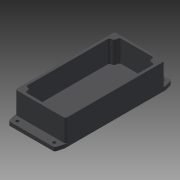
# Autodesk Inventor part: NEAMBoxLarge
Saved by Autodesk Inventor 2014 (Build 180170000, 170)
## iProperties
Created: 2015-04-18
Part Number: NEAMBoxLarge
Material: Generic
Document SubType Name: Modeling
Designer: Owner
Density: 1 g/cm^3
Appearance: Gray
Author: Owner
Autodesk Inventor part; units mm, degrees
ref_plane "YZ Plane" through (0, 0, 0) normal (1, 0, 0) x (0, 1, 0)
ref_plane "XZ Plane" through (0, 0, 0) normal (0, 1, 0) x (-1, 0, 0)
ref_plane "XY Plane" through (0, 0, 0) normal (0, 0, 1) x (1, 0, 0)
sketch "Sketch1" plane through (0, 0, 0) normal (0, 1, 0) x (-1, 0, 0)
  line L0 (-41.2899, 41.3823) -> (28.4387, 41.3823)
  line L1 (34.2779, 28.6823) -> (34.2779, -135.3255)
  line L2 (28.4387, -148.0255) -> (-41.2899, -148.0255)
  line L3 (-47.1291, -135.3255) -> (-47.1291, 28.6823)
  line L4 (-47.1291, 28.6823) -> (34.2779, 28.6823)
  line L5 (-47.1291, -135.3255) -> (34.2779, -135.3255)
  line L6 (34.2779, -135.3255) -> (31.5055, -145.6722)
  line L7 (-47.1291, -135.3255) -> (-44.3567, -145.6722)
  line L8 (-47.1291, 28.6823) -> (-44.3567, 39.0291)
  line L9 (34.2779, 28.6823) -> (31.5055, 39.0291)
  arc A0 (-44.3567, -145.6722) -> (-41.2899, -148.0255) centre (-41.2899, -144.8505) ccw
  arc A1 (28.4387, -148.0255) -> (31.5055, -145.6722) centre (28.4387, -144.8505) ccw
  arc A2 (31.5055, 39.0291) -> (28.4387, 41.3823) centre (28.4387, 38.2073) ccw
  arc A3 (-41.2899, 41.3823) -> (-44.3567, 39.0291) centre (-41.2899, 38.2073) ccw
  circle A4 centre (-36.423, -141.0151) radius 2.5019
  circle A5 centre (23.5718, -141.0151) radius 2.5019
  circle A6 centre (-36.423, 34.3719) radius 2.5019
  circle A7 centre (23.5718, 34.3719) radius 2.5019
  line L10 (-6.4256, 41.3823) -> (-6.4256, -148.0255) construction
  point P0 (0, 0)
  dimension "d2" = 12.7
  dimension "d3" = 12.7
  dimension "d4" = 15
  dimension "d5" = 15
  dimension "d6" = 15
  dimension "d7" = 81.407
  dimension "d8" = 189.4078
  dimension "d9" = 3.175
  dimension "d10" = 7.0104
  dimension "d11" = 7.0104
  dimension "d12" = 7.0104
  dimension "d13" = 7.0104
  dimension "d14" = 59.9948
  dimension "d15" = 59.9948
  dimension "d16" = 5.0038
  dimension "d17" = 5.0038
  dimension "d18" = 5.0038
  dimension "d19" = 5.0038
  dimension "d20" = 29.9974
  dimension "d21" = 29.9974
  constraints: 22 end point, 8 centre point, 8 point on circle, 8 tangent, 3 equal radius, 3 parallel, 3 perpendicular, 2 midpoint, 1 horizontal
  measures "d2" distance between parallel lines of L0 L4
  measures "d3" distance between parallel lines of L2 L5
  measures "d4" angle of L3 L8
  measures "d5" angle of L1 L9
  measures "d6" angle of L1 L6
  measures "d7" distance between parallel lines of L1 L3
  measures "d8" distance between parallel lines of L2 L0
  measures "d9" radius of A0
  measures "d10" distance from line of L0 A6.centre
  measures "d11" distance from line of L0 A7.centre
  measures "d12" distance from line of L2 A4.centre
  measures "d13" distance from line of L2 A5.centre
  measures "d14" distance of A5.centre A4.centre
  measures "d15" distance of A7.centre A6.centre
  measures "d16" diameter of A4
  measures "d17" diameter of A5
  measures "d18" diameter of A7
  measures "d19" diameter of A6
  measures "d20" distance from line of A7.centre L10
  measures "d21" distance from line of A5.centre L10
extrude "Extrusion1" add sketch "Sketch1" along normal blind 5.9944
sketch "Sketch2" plane through (0, 5.9944, 0) normal (0, 1, 0) x (1, 0, 0)
  line L0 (47.1291, -28.6823) -> (47.1291, 135.3255) projected
  line L1 (41.2899, 148.0255) -> (-28.4387, 148.0255) projected
  line L2 (-34.2779, 135.3255) -> (-34.2779, -28.6823) projected
  line L3 (-31.1029, 133.9285) -> (43.9541, 133.9285)
  line L4 (47.1291, 130.7535) -> (47.1291, -24.0849)
  line L5 (43.9541, -27.2599) -> (-31.1029, -27.2599)
  line L6 (-34.2779, -24.0849) -> (-34.2779, 130.7535)
  arc A0 (-34.2779, -24.0849) -> (-31.1029, -27.2599) centre (-31.1029, -24.0849) ccw
  arc A1 (43.9541, -27.2599) -> (47.1291, -24.0849) centre (43.9541, -24.0849) ccw
  arc A2 (47.1291, 130.7535) -> (43.9541, 133.9285) centre (43.9541, 130.7535) ccw
  arc A3 (-31.1029, 133.9285) -> (-34.2779, 130.7535) centre (-31.1029, 130.7535) ccw
  point P0 (0, 0)
  point P1 (-34.2779, 133.9285)
  point P2 (47.1291, -27.2599)
  dimension "d25" = 161.1884
  dimension "d26" = 14.097
  dimension "d27" = 3.175
  constraints: 8 end point, 8 point on circle, 8 tangent, 6 point on line, 4 centre point, 3 equal radius, 2 parallel, 1 horizontal, 1 perpendicular
  measures "d25" distance between parallel lines of L3 L5
  measures "d26" distance between parallel lines of L3 L1
  measures "d27" radius of A0
extrude "Extrusion2" add sketch "Sketch2" along normal blind 35.5092
sketch "Sketch3" plane through (0, 41.5036, 0) normal (0, 1, 0) x (1, 0, 0)
  line L0 (-34.2779, 130.7535) -> (-34.2779, -24.0849) projected
  line L1 (43.9541, 133.9285) -> (-31.1029, 133.9285) projected
  line L2 (42.9, 118.3456) -> (42.9, -11.2706)
  line L3 (-30.0488, -11.2706) -> (-30.0488, 118.3456)
  line L4 (-19.4443, 130.0169) -> (30.4413, 130.0169)
  line L5 (30.4413, -22.9419) -> (-19.4443, -22.9419)
  arc A0 (33.6163, 126.8419) -> (30.4413, 130.0169) centre (30.4413, 126.8419) ccw
  arc A1 (-19.4443, 130.0169) -> (-22.6193, 126.8419) centre (-19.4443, 126.8419) ccw
  arc A2 (-22.6193, -19.7669) -> (-19.4443, -22.9419) centre (-19.4443, -19.7669) ccw
  arc A3 (30.4413, -22.9419) -> (33.6163, -19.7669) centre (30.4413, -19.7669) ccw
  arc A4 (-30.0488, -11.2706) -> (-26.8738, -14.4456) centre (-26.8738, -11.2706) ccw
  arc A5 (-26.8738, 121.5206) -> (-30.0488, 118.3456) centre (-26.8738, 118.3456) ccw
  arc A6 (42.9, 118.3456) -> (39.725, 121.5206) centre (39.725, 118.3456) ccw
  arc A7 (39.725, -14.4456) -> (42.9, -11.2706) centre (39.725, -11.2706) ccw
  line L6 (33.6163, 126.8419) -> (33.6163, 126.0164)
  line L7 (33.6163, -18.9414) -> (33.6163, -19.7669)
  line L8 (-22.6193, -19.7669) -> (-22.6193, -18.9414)
  line L9 (-22.6193, 126.0164) -> (-22.6193, 126.8419)
  line L10 (39.725, -14.4456) -> (38.1121, -14.4456)
  line L11 (-27.1151, -14.4456) -> (-26.8738, -14.4456)
  line L12 (-26.8738, 121.5206) -> (-27.1151, 121.5206)
  line L13 (38.1121, 121.5206) -> (39.725, 121.5206)
  arc A8 (38.1121, -14.4456) -> (33.6163, -18.9414) centre (38.1121, -18.9414) ccw
  arc A9 (33.6163, 126.0164) -> (38.1121, 121.5206) centre (38.1121, 126.0164) ccw
  arc A10 (-27.1151, 121.5206) -> (-22.6193, 126.0164) centre (-27.1151, 126.0164) ccw
  arc A11 (-22.6193, -18.9414) -> (-27.1151, -14.4456) centre (-27.1151, -18.9414) ccw
  point P0 (0, 0)
  point P1 (42.9, 76.4991)
  point P2 (42.9, 110.1795)
  point P3 (-30.0488, 76.4991)
  point P4 (-22.7463, 130.0169)
  point P5 (33.6163, -22.9419)
  point P6 (33.6163, 130.0169)
  dimension "d30" = 56.3626
  dimension "d32" = 152.9588
  dimension "d35" = 72.9488
  dimension "d36" = 4.2291
  dimension "d37" = 3.9116
  dimension "d38" = 3.175
  dimension "d39" = 4.4958
  dimension "d42" = 135.9662
  dimension "d43" = 8.4963
  constraints: 32 tangent, 24 end point, 24 point on circle, 12 centre point, 10 equal radius, 10 parallel, 6 point on line, 4 perpendicular, 3 horizontal
  measures "d30" distance of point (-22.746, 130.017) point (33.616, 130.017)
  measures "d32" distance of point (33.616, 130.017) point (33.616, -22.942)
  measures "d35" distance of point (42.9, 76.499) point (-30.049, 76.499)
  measures "d36" distance between parallel lines of L0 L3
  measures "d37" distance between parallel lines of L1 L4
  measures "d38" radius of A0
  measures "d39" radius of A8
  measures "d42" distance between parallel lines of L13 L10
  measures "d43" distance between parallel lines of L13 L4
extrude "Extrusion3" cut sketch "Sketch3" against normal blind 35.5092
body "Solid1"
